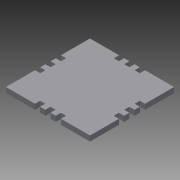
# Autodesk Inventor part: base
Saved by Autodesk Inventor 2014 SP1 (Build 180222100, 222)
## iProperties
Created: 2015-02-17
Part Number: base
Material: Generic
Document SubType Name: Modeling
Designer: Erin
Density: 1 g/cm^3
Appearance: Default
Author: Erin
Autodesk Inventor part; units mm, degrees
ref_plane "YZ Plane" through (0, 0, 0) normal (1, 0, 0) x (0, 1, 0)
ref_plane "XZ Plane" through (0, 0, 0) normal (0, 1, 0) x (-1, 0, 0)
ref_plane "XY Plane" through (0, 0, 0) normal (0, 0, 1) x (1, 0, 0)
sketch "slots" plane through (0, 0, 0) normal (0, 0, 1) x (1, 0, 0)
  line L0 (61.2067, 31.1821) -> (64.2567, 31.1821)
  line L1 (64.2567, 31.1821) -> (64.2567, 28.1071)
  line L2 (64.2567, 28.1071) -> (61.2067, 28.1071)
  line L3 (61.2067, 28.1071) -> (61.2067, 31.1821)
  line L4 (68.9317, 33.8834) -> (68.9317, 26.9198) construction
  line L5 (67.4067, 31.1821) -> (70.4567, 31.1821)
  line L6 (70.4567, 31.1821) -> (70.4567, 28.1071)
  line L7 (70.4567, 28.1071) -> (67.4067, 28.1071)
  line L8 (67.4067, 28.1071) -> (67.4067, 31.1821)
  line L9 (73.6067, 31.1821) -> (76.6567, 31.1821)
  line L10 (76.6567, 31.1821) -> (76.6567, 28.1071)
  line L11 (76.6567, 28.1071) -> (73.6067, 28.1071)
  line L12 (73.6067, 28.1071) -> (73.6067, 31.1821)
  line L13 (68.9317, 28.1071) -> (68.9317, 27.1937) construction
  point P0 (68.8645, 30.3856)
  dimension "d2" = 3.05
  dimension "d3" = 3.075
  dimension "d4" = 3.15
  dimension "d5" = 3.15
  measures "d2" distance of L1.end L2.end
  measures "d3" distance of L0.end L1.end
  measures "d4" distance between parallel lines of L8 L1
  measures "d5" distance between parallel lines of L12 L6
sketch "Sketch1" plane through (0, 0, 0) normal (0, 0, 1) x (1, 0, 0)
  line L0 (-25, 25) -> (25, 25)
  line L1 (25, 25) -> (25, -25)
  line L2 (25, -25) -> (-25, -25)
  line L3 (-25, -25) -> (-25, 25)
  line L4 (0, 40.2669) -> (0, -57.9846) construction
  line L5 (-45.3823, 0) -> (61.3149, 0) construction
  line L6 (-7.725, 25) -> (-4.675, 25)
  line L7 (-4.675, 25) -> (-4.675, 21.925)
  line L8 (-4.675, 21.925) -> (-7.725, 21.925)
  line L9 (-7.725, 21.925) -> (-7.725, 25)
  line L10 (0, 27.7013) -> (0, 20.7377) construction
  line L11 (-1.525, 25) -> (1.525, 25)
  line L12 (1.525, 25) -> (1.525, 21.925)
  line L13 (1.525, 21.925) -> (-1.525, 21.925)
  line L14 (-1.525, 21.925) -> (-1.525, 25)
  line L15 (4.675, 25) -> (7.725, 25)
  line L16 (7.725, 25) -> (7.725, 21.925)
  line L17 (7.725, 21.925) -> (4.675, 21.925)
  line L18 (4.675, 21.925) -> (4.675, 25)
  line L19 (0, 21.925) -> (0, 21.0116) construction
  line L20 (-7.725, -21.925) -> (-4.675, -21.925)
  line L21 (-4.675, -21.925) -> (-4.675, -25)
  line L22 (-4.675, -25) -> (-7.725, -25)
  line L23 (-7.725, -25) -> (-7.725, -21.925)
  line L24 (0, -19.2237) -> (0, -26.1873) construction
  line L25 (-1.525, -21.925) -> (1.525, -21.925)
  line L26 (1.525, -21.925) -> (1.525, -25)
  line L27 (1.525, -25) -> (-1.525, -25)
  line L28 (-1.525, -25) -> (-1.525, -21.925)
  line L29 (4.675, -21.925) -> (7.725, -21.925)
  line L30 (7.725, -21.925) -> (7.725, -25)
  line L31 (7.725, -25) -> (4.675, -25)
  line L32 (4.675, -25) -> (4.675, -21.925)
  line L33 (0, -25) -> (0, -25.9134) construction
  line L34 (-25, -7.725) -> (-25, -4.675)
  line L35 (-25, -4.675) -> (-21.925, -4.675)
  line L36 (-21.925, -4.675) -> (-21.925, -7.725)
  line L37 (-21.925, -7.725) -> (-25, -7.725)
  line L38 (-27.7013, 0) -> (-20.7377, 0) construction
  line L39 (-25, -1.525) -> (-25, 1.525)
  line L40 (-25, 1.525) -> (-21.925, 1.525)
  line L41 (-21.925, 1.525) -> (-21.925, -1.525)
  line L42 (-21.925, -1.525) -> (-25, -1.525)
  line L43 (-25, 4.675) -> (-25, 7.725)
  line L44 (-25, 7.725) -> (-21.925, 7.725)
  line L45 (-21.925, 7.725) -> (-21.925, 4.675)
  line L46 (-21.925, 4.675) -> (-25, 4.675)
  line L47 (-21.925, 0) -> (-21.0116, 0) construction
  line L48 (21.925, -7.725) -> (21.925, -4.675)
  line L49 (21.925, -4.675) -> (25, -4.675)
  line L50 (25, -4.675) -> (25, -7.725)
  line L51 (25, -7.725) -> (21.925, -7.725)
  line L52 (19.2237, 0) -> (26.1873, 0) construction
  line L53 (21.925, -1.525) -> (21.925, 1.525)
  line L54 (21.925, 1.525) -> (25, 1.525)
  line L55 (25, 1.525) -> (25, -1.525)
  line L56 (25, -1.525) -> (21.925, -1.525)
  line L57 (21.925, 4.675) -> (21.925, 7.725)
  line L58 (21.925, 7.725) -> (25, 7.725)
  line L59 (25, 7.725) -> (25, 4.675)
  line L60 (25, 4.675) -> (21.925, 4.675)
  line L61 (25, 0) -> (25.9134, 0) construction
  point P0 (0, 0)
  point P1 (25, 0)
  point P2 (0, 25)
  dimension "d0" = 50
  dimension "d1" = 50
  constraints: 12 end point, 6 horizontal, 5 vertical, 3 parallel, 2 midpoint, 2 perpendicular, 1 horizontal alignment, 1 vertical alignment
  measures "d0" distance of L1.end L2.end
  measures "d1" distance of L0.end L1.end
extrude "Extrusion1" add sketch "Sketch1" along normal blind 3.1 contours L0 L9 L8 L7 L14 L13 L12 L18 L17 L16 L1 L58 L57 L60 L54 L53 L56 L49 L48 L51 L2 L30 L29 L32 L26 L25 L28 L21 L20 L23 L3 L37 L36 L35 L42 L41 L40 L46 L45 L44
equation "\"d2\" = mat - kerf"
equation "\"d3\" = mat - 0.5 * kerf"
equation "\"d4\" = mat + kerf"
equation "\"d5\" = mat + kerf"
equation "\"d8\" = mat"
equation "\"mat\" = 3.1"
equation "\"kerf\" = 0.05"
body "Solid1"
